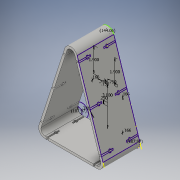
# Autodesk Inventor part: Nathan_LED_Speaker_Sides
Saved by Autodesk Inventor 2016 (Build 200138000, 138)
## iProperties
Created: 2018-09-27
Part Number: Nathan_LED_Speaker_Sides
Material: Generic
Document SubType Name: Modeling
Designer: Student
Density: 1 g/cm^3
Appearance: Default
Author: Student
Autodesk Inventor part; units mm, degrees
ref_plane "XZ Plane" through (0, 0, 0) normal (0, 1, 0) x (-1, 0, 0)
ref_plane "XY Plane" through (0, 0, 0) normal (0, 0, 1) x (1, 0, 0)
sketch "Sketch1" plane through (0, 0, 0) normal (0, 0, 1) x (1, 0, 0)
  arc A0 (0.6195, 16.618) -> (12.7, 0) centre (12.7, 12.7) ccw
  arc A1 (63.5, 182.0332) -> (51.4195, 173.2512) centre (63.5, 169.3332) ccw
  line L0 (0.6195, 16.618) -> (51.4195, 173.2512)
  arc A2 (114.3, 0) -> (126.3805, 16.618) centre (114.3, 12.7) ccw
  arc A3 (75.5805, 173.2512) -> (63.5, 182.0332) centre (63.5, 169.3332) ccw
  line L1 (126.3805, 16.618) -> (75.5805, 173.2512)
  line L2 (12.7, 0) -> (114.3, 0)
  arc A4 (71.2315, 171.8407) -> (55.7685, 171.8407) centre (63.5, 169.3332) ccw
  arc A5 (4.9685, 15.2075) -> (12.7, 4.572) centre (12.7, 12.7) ccw
  arc A6 (114.3, 4.572) -> (122.0315, 15.2075) centre (114.3, 12.7) ccw
  line L3 (4.9685, 15.2075) -> (55.7685, 171.8407)
  line L4 (114.3, 4.572) -> (12.7, 4.572)
  line L5 (122.0315, 15.2075) -> (71.2315, 171.8407)
  point P0 (0, 0)
  point P1 (0, 0)
  dimension "d1" = 12.7
  dimension "d2" = 12.7
  dimension "d3" = 12.7
  dimension "d4" = 101.6
  dimension "d6" = 72.031
  dimension "d10" = 164.6651
  dimension "d11" = 164.6651
  dimension "d23" = 16.256
  dimension "d24" = 4.572
  dimension "d25" = 16.256
  dimension "d26" = 16.256
  constraints: 14 point on circle, 12 end point, 7 centre point, 6 tangent, 2 coincident, 1 horizontal
  measures "d1" radius of A2
  measures "d2" radius of A3
  measures "d3" radius of A1
  measures "d4" distance of L2.start L2.end
  measures "d6" angle of L2 L0
  measures "d10" distance of L1.start L1.end
  measures "d11" distance of L0.start L0.end
  measures "d23" diameter of A4
  measures "d24" distance of L0.start L3.start
  measures "d25" diameter of A5
  measures "d26" diameter of A6
extrude "Extrusion1" add sketch "Sketch1" along normal blind 72.136
sketch "Sketch2" plane through (75.5805, 173.2512, 72.136) normal (0.9512, 0.3085, 0) x (0, 0, -1)
  line L0 (49.276, -155.7751) -> (49.276, -153.2351)
  line L1 (72.136, -153.2351) -> (72.136, -155.7751)
  line L2 (49.276, -8.89) -> (49.276, -11.43)
  line L3 (72.136, -11.43) -> (72.136, -8.89)
  line L4 (72.136, -164.6651) -> (0, -164.6651) projected
  line L5 (72.136, 0) -> (0, 0) projected
  line L6 (72.136, -83.6025) -> (72.136, -81.0625)
  line L7 (49.276, -83.6025) -> (49.276, -81.0625)
  line L8 (36.068, 0) -> (36.068, -164.6651)
  line L9 (72.136, -164.6651) -> (0, -164.6651) projected
  line L10 (54.1593, -82.3325) -> (54.1593, -79.4877)
  line L11 (54.1593, -83.6025) -> (54.1593, -85.1773)
  line L12 (54.1593, -85.1773) -> (56.7082, -85.1773)
  line L13 (56.7082, -79.4877) -> (54.1593, -79.4877)
  line L14 (72.136, -81.0625) -> (56.7082, -81.0625)
  line L15 (54.1593, -81.0625) -> (49.276, -81.0625)
  line L16 (49.276, -83.6025) -> (54.1593, -83.6025)
  line L17 (56.7082, -83.6025) -> (72.136, -83.6025)
  line L18 (56.7082, -85.1773) -> (56.7082, -83.6025)
  line L19 (56.7082, -81.0625) -> (56.7082, -79.4877)
  line L20 (54.1593, -153.2351) -> (54.1593, -151.6603)
  line L21 (54.1593, -157.3499) -> (56.7082, -157.3499)
  line L22 (56.7082, -151.6603) -> (54.1593, -151.6603)
  line L23 (56.7082, -157.3499) -> (56.7082, -155.7751)
  line L24 (56.7082, -153.2351) -> (56.7082, -151.6603)
  line L25 (54.1593, -157.3499) -> (54.1593, -154.5051)
  line L26 (54.1593, -8.89) -> (54.1593, -7.3152)
  line L27 (54.1593, -10.16) -> (54.1593, -13.0048)
  line L28 (54.1593, -13.0048) -> (56.7082, -13.0048)
  line L29 (56.7082, -7.3152) -> (54.1593, -7.3152)
  line L30 (56.7082, -13.0048) -> (56.7082, -11.43)
  line L31 (56.7082, -8.89) -> (56.7082, -7.3152)
  line L32 (22.86, -155.7751) -> (22.86, -153.2351)
  line L33 (0, -153.2351) -> (0, -155.7751)
  line L34 (22.86, -8.89) -> (22.86, -11.43)
  line L35 (0, -11.43) -> (0, -8.89)
  line L36 (0, -83.6025) -> (0, -81.0625)
  line L37 (22.86, -83.6025) -> (22.86, -81.0625)
  line L38 (17.9767, -82.3325) -> (17.9767, -79.4877)
  line L39 (17.9767, -83.6025) -> (17.9767, -85.1773)
  line L40 (17.9767, -85.1773) -> (15.4278, -85.1773)
  line L41 (15.4278, -79.4877) -> (17.9767, -79.4877)
  line L42 (0, -81.0625) -> (15.4278, -81.0625)
  line L43 (17.9767, -81.0625) -> (22.86, -81.0625)
  line L44 (22.86, -83.6025) -> (17.9767, -83.6025)
  line L45 (15.4278, -83.6025) -> (0, -83.6025)
  line L46 (15.4278, -85.1773) -> (15.4278, -83.6025)
  line L47 (15.4278, -81.0625) -> (15.4278, -79.4877)
  line L48 (17.9767, -153.2351) -> (17.9767, -151.6603)
  line L49 (17.9767, -157.3499) -> (15.4278, -157.3499)
  line L50 (15.4278, -151.6603) -> (17.9767, -151.6603)
  line L51 (15.4278, -157.3499) -> (15.4278, -155.7751)
  line L52 (15.4278, -153.2351) -> (15.4278, -151.6603)
  line L53 (17.9767, -157.3499) -> (17.9767, -154.5051)
  line L54 (17.9767, -8.89) -> (17.9767, -7.3152)
  line L55 (17.9767, -10.16) -> (17.9767, -13.0048)
  line L56 (17.9767, -13.0048) -> (15.4278, -13.0048)
  line L57 (15.4278, -7.3152) -> (17.9767, -7.3152)
  line L58 (15.4278, -13.0048) -> (15.4278, -11.43)
  line L59 (15.4278, -8.89) -> (15.4278, -7.3152)
  line L60 (22.86, -11.43) -> (17.9767, -11.43)
  line L61 (15.4278, -11.43) -> (0, -11.43)
  line L62 (0, -8.89) -> (15.4278, -8.89)
  line L63 (17.9767, -8.89) -> (22.86, -8.89)
  line L64 (72.136, -8.89) -> (56.7082, -8.89)
  line L65 (54.1593, -8.89) -> (49.276, -8.89)
  line L66 (49.276, -11.43) -> (54.1593, -11.43)
  line L67 (56.7082, -11.43) -> (72.136, -11.43)
  line L68 (49.276, -153.2351) -> (54.1593, -153.2351)
  line L69 (56.7082, -153.2351) -> (72.136, -153.2351)
  line L70 (72.136, -155.7751) -> (56.7082, -155.7751)
  line L71 (54.1593, -155.7751) -> (49.276, -155.7751)
  line L72 (22.86, -153.2351) -> (17.9767, -153.2351)
  line L73 (15.4278, -153.2351) -> (0, -153.2351)
  line L74 (0, -155.7751) -> (15.4278, -155.7751)
  line L75 (17.9767, -155.7751) -> (22.86, -155.7751)
  point P0 (72.136, -141.4835)
  point P1 (49.276, -82.3325)
  point P2 (22.86, -82.3325)
  dimension "d54" = 22.86
  dimension "d55" = 2.54
  dimension "d56" = 22.86
  dimension "d57" = 2.54
  dimension "d60" = 2.54
  dimension "d61" = 22.86
  dimension "d63" = 2.8448
  dimension "d64" = 2.8448
  dimension "d65" = 2.8448
  dimension "d66" = 2.8448
  dimension "d67" = 2.8448
  dimension "d68" = 2.8448
  dimension "d72" = 8.89
  dimension "d73" = 69.6325
  constraints: 146 end point, 38 symmetric about line, 26 perpendicular, 14 parallel, 6 horizontal, 6 point on line, 4 vertical, 2 midpoint
  measures "d54" distance of L1.end L0.start
  measures "d55" distance of L0.start L0.end
  measures "d56" distance of L3.end L2.start
  measures "d57" distance of L2.start L2.end
  measures "d60" distance of L6.end L6.start
  measures "d61" distance of L6.end L7.end
  measures "d63" distance of L10.start L10.end
  measures "d64" distance of L10.start L11.end
  measures "d65" distance of L25.end L20.end
  measures "d66" distance of L25.end L21.start
  measures "d67" distance of L27.start L26.end
  measures "d68" distance of L27.start L27.end
  measures "d72" distance between parallel lines of L4 L70
  measures "d73" distance between parallel lines of L69 L17
sketch "Sketch3" plane through (0, 0, 0) normal (0, 0, 1) x (1, 0, 0)
  line L0 (63.5, 50.8) -> (63.5, 44.45)
  circle A0 centre (63.5, 44.45) radius 38.1
  circle A1 centre (33.655, 74.295) radius 2.1082
  circle A2 centre (93.345, 74.295) radius 2.1082
  circle A3 centre (93.345, 14.605) radius 2.1082
  circle A4 centre (33.655, 14.605) radius 2.1082
  line L1 (63.5, 82.55) -> (63.5, 86.36)
  line L2 (63.5, 86.36) -> (82.55, 86.36)
  line L3 (63.5, 86.36) -> (44.45, 86.36)
  line L4 (82.55, 86.36) -> (82.55, 134.62)
  line L5 (44.45, 86.36) -> (44.45, 134.62)
  arc A5 (82.55, 134.62) -> (44.45, 134.62) centre (63.5, 134.62) ccw
  arc A6 (75.5805, 173.2512) -> (51.4195, 173.2512) centre (63.5, 169.3332) ccw projected
  circle A7 centre (63.5, 169.3332) radius 12.7
  line L6 (63.5, 169.3332) -> (75.5805, 173.2512)
  line L7 (63.5, 169.3332) -> (51.4195, 173.2512)
  arc A8 (114.3, 0) -> (126.3805, 16.618) centre (114.3, 12.7) ccw projected
  circle A9 centre (114.3, 12.7) radius 12.7
  line L8 (126.3805, 16.618) -> (114.3, 12.7)
  line L9 (114.3, 12.7) -> (114.3, 0)
  arc A10 (0.6195, 16.618) -> (12.7, 0) centre (12.7, 12.7) ccw projected
  circle A11 centre (12.7, 12.7) radius 12.7
  line L10 (12.7, 0) -> (12.7, 12.7)
  line L11 (12.7, 12.7) -> (0.6195, 16.618)
  dimension "d42" = 76.2
  dimension "d41" = 6.35
  dimension "d43" = 4.2164
  dimension "d44" = 4.2164
  dimension "d45" = 4.2164
  dimension "d46" = 4.2164
  dimension "d47" = 3.81
  dimension "d48" = 19.05
  dimension "d49" = 19.05
  dimension "d50" = 48.26
  dimension "d51" = 48.26
  dimension "d74" = 144.062
  dimension "d75" = 107.969
  dimension "d76" = 107.969
  constraints: 24 end point, 6 centre point, 6 vertical, 4 coincident, 2 horizontal, 2 point on circle, 1 vertical alignment, 8 other
  measures "d41" distance of L0.start L0.end
  measures "d43" diameter of A1
  measures "d44" diameter of A2
  measures "d45" diameter of A3
  measures "d46" diameter of A4
  measures "d47" distance of L1.start L1.end
  measures "d48" distance of L1.end L2.end
  measures "d49" distance of L1.end L3.end
  measures "d50" distance of L2.end L4.end
  measures "d51" distance of L3.end L5.end
  measures "d74" angle of L7 L6
  measures "d75" angle of L9 L8
  measures "d76" angle of L10 L11
extrude "Extrusion2" cut sketch "Sketch2" against normal blind 25.4
ref_plane "Work Plane1" through (63.5, 0, 0) normal (1, 0, 0) x (0, 1, 0)
mirror "Mirror1" about plane through (63.5, 0, 0) normal (1, 0, 0) of "Extrusion2"
sketch "Sketch5" plane through (126.3805, 16.618, 72.136) normal (0.9512, 0.3085, 0) x (0, 0, -1)
  line L0 (72.136, 164.6651) -> (0, 164.6651) projected
  line L1 (72.136, 0) -> (0, 0) projected
  line L2 (0, 164.6651) -> (72.136, 164.6651)
  line L3 (72.136, 164.6651) -> (72.136, 0)
  line L4 (72.136, 0) -> (0, 0)
  line L5 (0, 0) -> (0, 164.6651)
  line L6 (15.4278, 155.7751) -> (0, 155.7751) projected
  line L7 (0, 155.7751) -> (15.4278, 155.7751)
  line L8 (17.9767, 157.3499) -> (15.4278, 157.3499) projected
  line L9 (15.4278, 155.7751) -> (15.4278, 157.3499)
  line L10 (15.4278, 157.3499) -> (17.9767, 157.3499)
  line L11 (17.9767, 157.3499) -> (17.9767, 155.7751)
  line L12 (22.86, 155.7751) -> (17.9767, 155.7751) projected
  line L13 (17.9767, 155.7751) -> (22.86, 155.7751)
  line L14 (22.86, 155.7751) -> (22.86, 153.2351) projected
  line L15 (22.86, 155.7751) -> (22.86, 153.2351)
  line L16 (17.9767, 151.6603) -> (17.9767, 153.2351) projected
  line L17 (22.86, 153.2351) -> (17.9767, 153.2351)
  line L18 (17.9767, 153.2351) -> (17.9767, 151.6603)
  line L19 (17.9767, 151.6603) -> (15.4278, 151.6603) projected
  line L20 (17.9767, 151.6603) -> (15.4278, 151.6603)
  line L21 (15.4278, 153.2351) -> (15.4278, 151.6603) projected
  line L22 (15.4278, 151.6603) -> (15.4278, 153.2351)
  line L23 (0, 153.2351) -> (0, 83.6025) projected
  line L24 (15.4278, 153.2351) -> (0, 153.2351)
  line L25 (0, 83.6025) -> (15.4278, 83.6025)
  line L26 (17.9767, 85.1773) -> (15.4278, 85.1773) projected
  line L27 (15.4278, 83.6025) -> (15.4278, 85.1773)
  line L28 (15.4278, 85.1773) -> (17.9767, 85.1773)
  line L29 (17.9767, 83.6025) -> (17.9767, 85.1773) projected
  line L30 (17.9767, 85.1773) -> (17.9767, 83.6025)
  line L31 (22.86, 83.6025) -> (17.9767, 83.6025) projected
  line L32 (17.9767, 83.6025) -> (22.86, 83.6025)
  line L33 (22.86, 83.6025) -> (22.86, 81.0625) projected
  line L34 (22.86, 83.6025) -> (22.86, 81.0625)
  line L35 (17.9767, 81.0625) -> (22.86, 81.0625) projected
  line L36 (22.86, 81.0625) -> (17.9767, 81.0625)
  line L37 (17.9767, 79.4877) -> (17.9767, 81.0625) projected
  line L38 (17.9767, 81.0625) -> (17.9767, 79.4877)
  line L39 (15.4278, 79.4877) -> (17.9767, 79.4877) projected
  line L40 (17.9767, 79.4877) -> (15.4278, 79.4877)
  line L41 (15.4278, 79.4877) -> (15.4278, 81.0625) projected
  line L42 (15.4278, 79.4877) -> (15.4278, 81.0625)
  line L43 (15.4278, 81.0625) -> (0, 81.0625)
  line L44 (0, 104.4301) -> (0, 48.0522) projected
  line L45 (0, -7.7315) -> (0, 23.6126) projected
  line L46 (15.4278, 8.89) -> (15.4278, 7.3152) projected
  line L47 (0, 8.89) -> (15.4278, 8.89)
  line L48 (15.4278, 8.89) -> (15.4278, 7.3152)
  line L49 (15.4278, 7.3152) -> (17.9767, 7.3152)
  line L50 (22.86, 8.89) -> (17.9767, 8.89) projected
  line L51 (17.9767, 8.89) -> (22.86, 8.89)
  line L52 (22.86, 11.43) -> (22.86, 8.89) projected
  line L53 (22.86, 8.89) -> (22.86, 11.43)
  line L54 (22.86, 11.43) -> (17.9767, 11.43)
  line L55 (17.9767, 11.43) -> (17.9767, 13.0048) projected
  line L56 (17.9767, 11.43) -> (17.9767, 13.0048)
  line L57 (17.9767, 13.0048) -> (15.4278, 13.0048)
  line L58 (15.4278, 13.0048) -> (15.4278, 11.43)
  line L59 (72.136, 19.2636) -> (72.136, -12.0805) projected
  line L60 (72.136, 8.89) -> (56.7082, 8.89) projected
  line L61 (72.136, 8.89) -> (56.7082, 8.89)
  line L62 (54.1593, 7.3152) -> (56.7082, 7.3152) projected
  line L63 (56.7082, 8.89) -> (56.7082, 7.3152)
  line L64 (56.7082, 7.3152) -> (54.1593, 7.3152)
  line L65 (54.1593, 8.89) -> (54.1593, 7.3152) projected
  line L66 (54.1593, 7.3152) -> (54.1593, 8.89)
  line L67 (49.276, 8.89) -> (49.276, 11.43) projected
  line L68 (54.1593, 8.89) -> (49.276, 8.89)
  line L69 (49.276, 8.89) -> (49.276, 11.43)
  line L70 (49.276, 11.43) -> (54.1593, 11.43) projected
  line L71 (49.276, 11.43) -> (54.1593, 11.43)
  line L72 (54.1593, 11.43) -> (54.1593, 13.0048) projected
  line L73 (54.1593, 11.43) -> (54.1593, 13.0048)
  line L74 (54.1593, 13.0048) -> (56.7082, 13.0048) projected
  line L75 (54.1593, 13.0048) -> (56.7082, 13.0048)
  line L76 (56.7082, 13.0048) -> (56.7082, 11.43) projected
  line L77 (56.7082, 13.0048) -> (56.7082, 11.43)
  line L78 (56.7082, 11.43) -> (72.136, 11.43)
  line L79 (72.136, 101.7468) -> (72.136, 45.3688) projected
  line L80 (56.7082, 81.0625) -> (56.7082, 79.4877) projected
  line L81 (72.136, 81.0625) -> (56.7082, 81.0625)
  line L82 (56.7082, 81.0625) -> (56.7082, 79.4877)
  line L83 (54.1593, 81.0625) -> (54.1593, 79.4877) projected
  line L84 (56.7082, 79.4877) -> (54.1593, 79.4877)
  line L85 (54.1593, 79.4877) -> (54.1593, 81.0625)
  line L86 (49.276, 81.0625) -> (49.276, 83.6025) projected
  line L87 (54.1593, 81.0625) -> (49.276, 81.0625)
  line L88 (49.276, 81.0625) -> (49.276, 83.6025)
  line L89 (49.276, 83.6025) -> (54.1593, 83.6025) projected
  line L90 (49.276, 83.6025) -> (54.1593, 83.6025)
  line L91 (54.1593, 85.1773) -> (54.1593, 83.6025) projected
  line L92 (54.1593, 83.6025) -> (54.1593, 85.1773)
  line L93 (56.7082, 85.1773) -> (54.1593, 85.1773) projected
  line L94 (54.1593, 85.1773) -> (56.7082, 85.1773)
  line L95 (56.7082, 83.6025) -> (56.7082, 85.1773) projected
  line L96 (56.7082, 85.1773) -> (56.7082, 83.6025)
  line L97 (56.7082, 83.6025) -> (72.136, 83.6025)
  line L98 (72.136, 160.1812) -> (72.136, 103.8033) projected
  line L99 (56.7082, 153.2351) -> (72.136, 153.2351) projected
  line L100 (72.136, 153.2351) -> (56.7082, 153.2351)
  line L101 (56.7082, 151.6603) -> (56.7082, 153.2351) projected
  line L102 (56.7082, 153.2351) -> (56.7082, 151.6603)
  line L103 (54.1593, 151.6603) -> (56.7082, 151.6603) projected
  line L104 (56.7082, 151.6603) -> (54.1593, 151.6603)
  line L105 (54.1593, 151.6603) -> (54.1593, 153.2351) projected
  line L106 (54.1593, 151.6603) -> (54.1593, 153.2351)
  line L107 (49.276, 155.7751) -> (49.276, 153.2351) projected
  line L108 (54.1593, 153.2351) -> (49.276, 153.2351)
  line L109 (49.276, 153.2351) -> (49.276, 155.7751)
  line L110 (54.1593, 155.7751) -> (49.276, 155.7751) projected
  line L111 (49.276, 155.7751) -> (54.1593, 155.7751)
  line L112 (56.7082, 157.3499) -> (54.1593, 157.3499) projected
  line L113 (54.1593, 155.7751) -> (54.1593, 157.3499)
  line L114 (54.1593, 157.3499) -> (56.7082, 157.3499)
  line L115 (72.136, 155.7751) -> (56.7082, 155.7751) projected
  line L116 (56.7082, 157.3499) -> (56.7082, 155.7751)
  line L117 (56.7082, 155.7751) -> (72.136, 155.7751)
  line L118 (15.4278, 7.3152) -> (17.9767, 7.3152) projected
  line L119 (17.9767, 7.3152) -> (17.9767, 8.89)
  line L120 (15.4278, 11.43) -> (0, 11.43) projected
  line L121 (15.4278, 11.43) -> (0, 11.43)
  point P0 (72.136, 23.1816)
  constraints: 140 end point, 43 perpendicular, 17 equal length, 12 point on line, 4 horizontal, 3 vertical
sketch "Sketch6" plane through (12.7, 0, 0) normal (0, -1, 0) x (1, 0, 0)
  line L0 (3.81, 0) -> (3.81, 15.4178)
  line L1 (3.81, 15.4178) -> (2.2352, 15.4178)
  line L2 (2.2352, 15.4178) -> (2.2352, 17.9578)
  line L3 (2.2352, 17.9578) -> (3.81, 17.9578)
  line L4 (3.81, 17.9578) -> (3.81, 22.8346)
  line L5 (3.81, 22.8346) -> (6.35, 22.8346)
  line L6 (6.35, 22.8346) -> (6.35, 17.9578)
  line L7 (6.35, 17.9578) -> (7.9248, 17.9578)
  line L8 (7.9248, 17.9578) -> (7.9248, 15.4178)
  line L9 (7.9248, 15.4178) -> (6.35, 15.4178)
  line L10 (6.35, 15.4178) -> (6.35, 0)
  line L11 (101.6, 0) -> (101.6, 72.136) projected
  line L12 (0, 0) -> (101.6, 0) projected
  line L13 (97.79, 0) -> (97.79, 15.4178)
  line L14 (97.79, 0) -> (113.2078, 0) construction
  line L15 (97.79, 15.4178) -> (99.3648, 15.4178)
  line L16 (99.3648, 15.4178) -> (99.3648, 17.9578)
  line L17 (99.3648, 17.9578) -> (97.79, 17.9578)
  line L18 (97.79, 17.9578) -> (97.79, 22.8346)
  line L19 (97.79, 22.8346) -> (95.2505, 22.8346)
  line L20 (95.2505, 22.8346) -> (95.2505, 17.9578)
  line L21 (95.2505, 17.9578) -> (93.6757, 17.9578)
  line L22 (93.6757, 17.9578) -> (93.6757, 15.4178)
  line L23 (93.6757, 15.4178) -> (95.2505, 15.4178)
  line L24 (95.2505, 15.4178) -> (95.2505, 0)
  line L25 (0, 0) -> (0, 72.136) projected
  line L26 (3.81, 72.136) -> (3.81, 56.7182)
  line L27 (3.81, 56.7182) -> (2.2352, 56.7182)
  line L28 (2.2352, 56.7182) -> (2.2352, 54.1782)
  line L29 (2.2352, 54.1782) -> (3.81, 54.1782)
  line L30 (3.81, 54.1782) -> (3.81, 49.3014)
  line L31 (3.81, 49.3014) -> (6.35, 49.3014)
  line L32 (6.35, 49.3014) -> (6.35, 54.1782)
  line L33 (6.35, 54.1782) -> (7.9248, 54.1782)
  line L34 (7.9248, 54.1782) -> (7.9248, 56.7182)
  line L35 (7.9248, 56.7182) -> (6.35, 56.7182)
  line L36 (6.35, 56.7182) -> (6.35, 72.136)
  line L37 (97.79, 72.136) -> (97.79, 56.7182)
  line L38 (97.79, 56.7182) -> (99.3648, 56.7182)
  line L39 (99.3648, 56.7182) -> (99.3648, 54.1782)
  line L40 (99.3648, 54.1782) -> (97.79, 54.1782)
  line L41 (97.79, 54.1782) -> (97.79, 49.3014)
  line L42 (97.79, 49.3014) -> (95.2505, 49.3014)
  line L43 (95.2505, 49.3014) -> (95.2505, 54.1782)
  line L44 (95.2505, 54.1782) -> (93.6757, 54.1782)
  line L45 (93.6757, 54.1782) -> (93.6757, 56.7182)
  line L46 (93.6757, 56.7182) -> (95.2505, 56.7182)
  line L47 (95.2505, 56.7182) -> (95.2505, 72.136)
  line L48 (0, 72.136) -> (101.6, 72.136) projected
  line L49 (0, 72.136) -> (101.6, 72.136)
  line L50 (0, 0) -> (101.6, 0)
  line L51 (0, 72.136) -> (0, 0)
  line L52 (101.6, 0) -> (101.6, 72.136)
  line L53 (3.81, 0) -> (6.35, 0)
  line L54 (3.81, 72.136) -> (6.35, 72.136)
  line L55 (95.2505, 72.136) -> (97.79, 72.136)
  point P0 (-12.7, 0)
  dimension "d78" = 15.4178
  dimension "d79" = 1.5748
  dimension "d80" = 2.54
  dimension "d81" = 4.8768
  dimension "d82" = 2.54
  dimension "d83" = 1.5748
  dimension "d86" = 15.4178
  dimension "d87" = 90
  dimension "d88" = 1.5748
  dimension "d89" = 1.5748
  dimension "d90" = 15.4178
  dimension "d91" = 3.81
  dimension "d92" = 17.9578
  dimension "d93" = 17.9578
  dimension "d94" = 15.4178
  dimension "d96" = 17.9578
  dimension "d97" = 5.6891
  dimension "d98" = 3.81
  dimension "d99" = 3.81
  dimension "d100" = 22.8346
  dimension "d101" = 15.4178
  dimension "d102" = 15.4178
  dimension "d103" = 4.8768
  dimension "d104" = 4.8768
  dimension "d105" = 2.54
  dimension "d106" = 1.5748
  dimension "d107" = 1.5748
  dimension "d108" = 2.54
  dimension "d109" = 2.54
  dimension "d110" = 1.5748
  dimension "d111" = 1.5748
  dimension "d112" = 2.54
  dimension "d113" = 5.6896
  dimension "d114" = 15.4178
  dimension "d115" = 17.9578
  dimension "d116" = 88.9005
  dimension "d117" = 85.7509
  dimension "d118" = 2.5395
  dimension "d119" = 15.4178
  dimension "d120" = 15.4178
  dimension "d121" = 2.54
  dimension "d122" = 2.54
  dimension "d123" = 2.5395
  dimension "d124" = 4.8768
  dimension "d125" = 4.8768
  dimension "d126" = 1.5748
  dimension "d127" = 1.5748
  dimension "d128" = 5.6891
  dimension "d129" = 2.5395
  constraints: 104 end point, 22 point on line, 16 perpendicular, 4 horizontal, 2 collinear, 1 vertical
  measures "d78" distance of L0.start L0.end
  measures "d79" distance of L0.end L1.end
  measures "d80" distance of L1.end L2.end
  measures "d81" distance of L3.end L4.end
  measures "d82" distance of L4.end L5.end
  measures "d83" distance of L6.end L7.end
  measures "d86" distance of L13.start L13.end
  measures "d87" angle of L14 L13
  measures "d88" distance of L13.end L15.end
  measures "d89" distance of L20.end L21.end
  measures "d90" distance of L9.end L10.end
  measures "d91" distance between parallel lines of L25 L0
  measures "d92" distance between parallel lines of L50 L3
  measures "d93" distance between parallel lines of L50 L7
  measures "d94" distance between parallel lines of L12 L9
  measures "d96" distance between parallel lines of L12 L17
  measures "d97" distance between parallel lines of L16 L22
  measures "d98" distance between parallel lines of L11 L13
  measures "d99" distance between parallel lines of L11 L18
  measures "d100" distance between parallel lines of L12 L19
  measures "d101" distance of L35.end L36.end
  measures "d102" distance of L26.start L27.start
  measures "d103" distance of L31.end L33.start
  measures "d104" distance of L30.start L31.start
  measures "d105" distance of L31.start L31.end
  measures "d106" distance of L33.start L33.end
  measures "d107" distance of L29.start L30.start
  measures "d108" distance of L28.start L29.start
  measures "d109" distance of L33.end L35.start
  measures "d110" distance of L35.start L35.end
  measures "d111" distance of L27.start L28.start
  measures "d112" distance between parallel lines of L36 L26
  measures "d113" distance between parallel lines of L34 L28
  measures "d114" distance between parallel lines of L49 L35
  measures "d115" distance between parallel lines of L49 L33
  measures "d116" distance between parallel lines of L47 L36
  measures "d117" distance between parallel lines of L45 L34
  measures "d118" distance between parallel lines of L37 L47
  measures "d119" distance of L46.end L47.end
  measures "d120" distance of L37.start L38.start
  measures "d121" distance of L45.start L45.end
  measures "d122" distance of L38.end L39.end
  measures "d123" distance of L41.end L43.start
  measures "d124" distance of L41.start L41.end
  measures "d125" distance of L43.start L44.start
  measures "d126" distance of L38.start L38.end
  measures "d127" distance of L39.end L41.start
  measures "d128" distance between parallel lines of L39 L45
  measures "d129" distance between parallel lines of L41 L43
extrude "Extrusion3" cut sketch "Sketch6" against normal blind 25.4 contours L0 L1 L2 L3 L4 L5 L6 L7 L8 L9 L10 L12 | L24 L23 L22 L21 L20 L19 L18 L17 L16 L15 L13 L12 | L48 L36 L35 L34 L33 L32 L31 L30 L29 L28 L27 L26 | L48 L37 L38 L39 L40 L41 L42 L43 L44 L45 L46 L47
body "Solid1"
